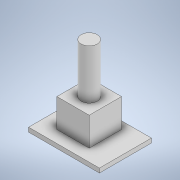
# Autodesk Inventor part: Rotary_Encoder_Model
Saved by Autodesk Inventor 2021 (Build 250183000, 183)
## iProperties
Created: 2020-07-08
Part Number: Rotary_Encoder_Model
Material: Generic
Document SubType Name: Modeling
Designer: ameli
Density: 1 g/cm^3
Appearance: Default
Author: ameli
Autodesk Inventor part; units mm, degrees
ref_plane "YZ Plane" through (0, 0, 0) normal (1, 0, 0) x (0, 1, 0)
ref_plane "XZ Plane" through (0, 0, 0) normal (0, 1, 0) x (-1, 0, 0)
ref_plane "XY Plane" through (0, 0, 0) normal (0, 0, 1) x (1, 0, 0)
sketch "Sketch1" plane through (0, 0, 0) normal (0, 1, 0) x (-1, 0, 0)
  line L0 (13.15, 9.65) -> (-13.15, 9.65)
  line L1 (-13.15, 9.65) -> (-13.15, -9.65)
  line L2 (-13.15, -9.65) -> (13.15, -9.65)
  line L3 (13.15, -9.65) -> (13.15, 9.65)
  point P0 (0, 0)
  dimension "d0" = 19.3
  dimension "d1" = 26.3
  dimension "d2" = 9.65
  dimension "d3" = 13.15
  constraints: 8 end point, 2 parallel, 1 horizontal, 1 perpendicular
  measures "d0" distance of L0.end L1.end
  measures "d1" distance of L1.end L2.end
  measures "d2" distance from line of point (0, 0) L2
  measures "d3" distance from line of point (0, 0) L1
extrude "Extrusion1" add sketch "Sketch1" along normal blind 1.6
sketch "Sketch2" plane through (0, 1.6, 0) normal (0, 1, 0) x (1, 0, 0)
  line L0 (-7.15, -5.15) -> (4.85, -5.15)
  line L1 (4.85, -5.15) -> (4.85, 6.85)
  line L2 (4.85, 6.85) -> (-7.15, 6.85)
  line L3 (-7.15, 6.85) -> (-7.15, -5.15)
  line L4 (13.15, 9.65) -> (-13.15, 9.65) projected
  line L5 (-13.15, 9.65) -> (-13.15, -9.65) projected
  point P0 (0, 0)
  dimension "d6" = 12
  dimension "d7" = 12
  dimension "d8" = 2.8
  dimension "d9" = 6
  constraints: 8 end point, 2 parallel, 1 horizontal, 1 perpendicular
  measures "d6" distance of L2.end L0.start
  measures "d7" distance of L1.end L2.end
  measures "d8" distance between parallel lines of L4 L2
  measures "d9" distance between parallel lines of L5 L3
extrude "Extrusion2" add sketch "Sketch2" along normal blind 10.6
sketch "Sketch3" plane through (0, 12.2, 0) normal (0, 1, 0) x (1, 0, 0)
  circle A0 centre (-1.15, 0.85) radius 3
  line L0 (-7.15, 6.85) -> (-7.15, -5.15) projected
  line L1 (4.85, 6.85) -> (-7.15, 6.85) projected
  point P0 (0, 0)
  dimension "d12" = 6
  dimension "d13" = 6
  dimension "d14" = 6
  constraints: 1 centre point
  measures "d12" diameter of A0
  measures "d13" distance from line of L0 A0.centre
  measures "d14" distance from line of L1 A0.centre
extrude "Extrusion3" add sketch "Sketch3" along normal blind 18.4
body "Solid1"
